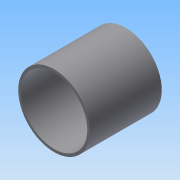
# Autodesk Inventor part: verre
Saved by Autodesk Inventor 2013 (Build 170138000, 138)
## iProperties
Created: 2012-11-14
Part Number: verre
Material: Générique
Document SubType Name: Modeling
Designer: Aegir
Density: 1 g/cm^3
Author: Aegir
Autodesk Inventor part; units mm, degrees
ref_plane "YZ Plane" through (0, 0, 0) normal (1, 0, 0) x (0, 1, 0)
ref_plane "XZ Plane" through (0, 0, 0) normal (0, 1, 0) x (-1, 0, 0)
ref_plane "XY Plane" through (0, 0, 0) normal (0, 0, 1) x (1, 0, 0)
sketch "Esquisse1" plane through (0, 0, 0) normal (0, 1, 0) x (-1, 0, 0)
  circle A0 centre (0, 0) radius 40
  circle A1 centre (0, 0) radius 37
  dimension "d0" = 74
  dimension "d2" = 80
  constraints: 2 centre point, 2 coincident
  measures "d0" diameter of A1
  measures "d2" diameter of A0
extrude "Extrusion1" add sketch "Esquisse1" along normal blind 80
sketch "Esquisse2" plane through (0, 80, 0) normal (0, 1, 0) x (1, 0, 0)
  circle A0 centre (0, 0) radius 37 projected
  circle A1 centre (0, 0) radius 40 projected
  circle A2 centre (0, 0) radius 37
  constraints: 1 centre point, 1 coincident, 1 concentric
extrude "Extrusion2" add sketch "Esquisse2" against normal blind 5 contours A0
